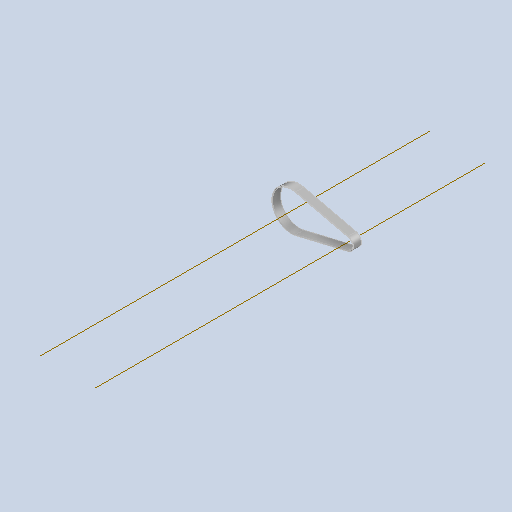
# Autodesk Inventor part: Synchronous Belt
Saved by Autodesk Inventor 2023 (Build 270158000, 158)
## iProperties
CustomPartVersion: 1
Created: 2022-01-04
Part Number: Synchronous Belt
Material: Rubber
Document SubType Name: Modeling
Designer: Jochen
Density: 1 g/cm^3
Appearance: Rubber - Black - Version 1.1
Author: Jochen
Autodesk Inventor part; units mm, degrees
sketch "Sketch Path" plane through (0, 0, 0) normal (0, 0, 1) x (1, 0, 0)
  arc A0 (1.1015, -4.6459) -> (1.1015, 4.6459) centre (0, 0) ccw
  arc A1 (-38.0891, 13.9376) -> (-38.0891, -13.9376) centre (-41.3935, 0) ccw
  line L0 (-38.0891, 13.9376) -> (1.1015, 4.6459)
  line L1 (1.1015, -4.6459) -> (-38.0891, -13.9376)
  constraints: 4 end point, 4 point on circle, 2 centre point
ref_plane "Cross Section Plane" through (1.1015, 4.6459, 0) normal (-0.973, 0.2307, 0) x (0, 0, 1)
ref_plane "Work Plane2" through (0, 0, 0) normal (-1, 0, 0) x (0, 0, 1)
ref_plane "Work Plane3" through (-41.3935, 0, 0) normal (0.9848, 0.1736, 0) x (0, 0, 1)
sketch "Cross Section" plane through (1.1015, 4.6459, 0) normal (-0.973, 0.2307, 0) x (0, 0, 1)
  line L0 (-3, 0.3) -> (3, 0.3)
  line L1 (3, 0.3) -> (3, -0.3)
  line L2 (3, -0.3) -> (-3, -0.3)
  line L3 (-3, -0.3) -> (-3, 0.3)
  line L4 (-3, 0) -> (3, 0) construction
  point P0 (0, 0)
  point P1 (0, 0)
  dimension "d0" = 6
  dimension "d4" = 0.3
  dimension "d5" = 0.3
  constraints: 10 end point, 3 midpoint, 2 parallel, 1 coincident, 1 horizontal, 1 perpendicular, 1 other
  measures "d0" distance between parallel lines of L1 L3
  measures "d4" distance between parallel lines of L2 L4
  measures "d5" distance between parallel lines of L4 L0
sweep "Belt" add profiles "Cross Section" path "Sketch Path"
equation "\"d0\" = da_B"
equation "\"d4\" = da_a"
equation "\"d5\" = da_a2"
equation "\"da_B\" = 6"
equation "\"da_pb\" = 2.5"
equation "\"da_L\" = 145"
equation "\"da_a\" = 0.3"
equation "\"da_S\" = 1.5"
equation "\"da_Beta\" = 20deg"
equation "\"da_Ht\" = 0.7"
equation "\"da_H\" = 1.3"
equation "\"da_a2\" = 0.3"
body "Solid1"
